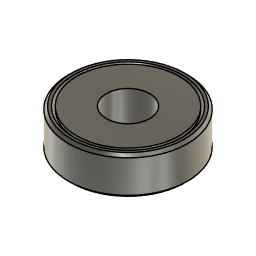
Full Assembly (Autodesk Fusion 360 archive; units mm, degrees)
design "Assembly_Bearing"
Autodesk Fusion 360 part; units mm, degrees
sketch "Sketch1" plane through (0, 0, 0) normal (0, 0, 1) x (1, 0, 0)
  circle A0 centre (0, 0) radius 4
  circle A1 centre (0, 0) radius 11
  dimension "d93" = 8
  dimension "d94" = 22
  constraint coincident A0.centre A1.centre
  measures "d93" diameter of A0
  measures "d94" diameter of A1
extrude "Extrude1" add sketch "Sketch1" along normal blind 7 makes body 1
move_face "OffsetFaces2" offset -1.5 1 faces at (10.9453, -1.0952, 4.6667) on bodies 1
sketch "Sketch2" plane through (0, 0, 0) normal (1, 0, 0) x (0, 1, 0)
  line L0 (9.5, 7) -> (-9.5, 7)
  line L1 (9.5, 0) -> (-9.5, 0)
  line L2 (9.5, 7) -> (11, 7)
  line L3 (11, 7) -> (11, 0)
  line L4 (11, 0) -> (9.5, 0)
  line L5 (9.5, 0) -> (9.5, 7)
  line L6 (-4, 0) -> (4, 0)
  line L7 (9.5, 0) -> (-9.5, 0)
  dimension "d98" = 1.5
  constraint horizontal L2
  constraint vertical L3
  constraint horizontal L4
  constraint vertical L5
  constraint coincident L0.start L2.start
  constraint coincident L4 L1.start
  measures "d98" distance of L0.start L2.end
revolve "Revolve1" add sketch "Sketch2" angle 360 about axis through (0, 0, 0) along (0, 0, -1) separate body makes body 2
chamfer "Chamfer1" distance 0.5 angle 45 4 edges at (-10.2556, 3.9778, 7) (-8.8571, 3.4353, 7) (-10.2556, 3.9778, 0) (-8.8571, 3.4353, 0) on bodies 2
copy_body "Body->Comp1" bodies 1 removing the originals makes body 3 in component "Inner"
copy_body "Body->Comp2" bodies 2 removing the originals makes body 4 in component "Outer"
hole "Hole1" at (-11, 0, 3.0079) direction (1, 0, 0) diameter 2 depth 1 tip angle 180 bodies 4 in component "Outer"
component "Inner" placed x (1, 0, 0) y (0, 1, 0) z (0, 0, 1) at (0, 0, 0)
component "Outer" placed x (1, 0, 0) y (0, 1, 0) z (0, 0, 1) at (0, 0, 0)
